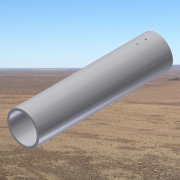
# Autodesk Inventor part: hub-sleeve
Saved by Autodesk Inventor 2013 (Build 170138000, 138)
## iProperties
Company: HERA Project
Created: 2013-05-14
Part Number: hub-sleeve
Material: PVC-Piping
Document SubType Name: Modeling
Designer: David DeBoer
Density: 1.4 g/cm^3
Mass: 429.807 g
Surface Area: 1214.86 cm^2
Volume: 307.005 cm^3
Description: Hub mating sleeve
Author: David DeBoer
Title: Hub mating sleeve
Autodesk Inventor part; units mm, degrees
ref_plane "YZ Plane" through (0, 0, 0) normal (1, 0, 0) x (0, 1, 0)
ref_plane "XZ Plane" through (0, 0, 0) normal (0, 1, 0) x (-1, 0, 0)
ref_plane "XY Plane" through (0, 0, 0) normal (0, 0, 1) x (1, 0, 0)
sketch "Sketch1" plane through (0, 0, 0) normal (0, 0, 1) x (1, 0, 0)
  circle A0 centre (0, 0) radius 36.5125
  circle A1 centre (0, 0) radius 31.3563
  dimension "d0" = 73.025
  dimension "d2" = 5.1562
  constraints: 2 centre point, 1 coincident
  measures "d0" diameter of A0
  measures "d2" radial gap between concentric circles of A1 A0
extrude "Extrusion1" add sketch "Sketch1" along normal blind 304.8
sketch "Sketch2" plane through (0, 0, 304.8) normal (0, 0, 1) x (1, 0, 0)
  circle A0 centre (0, 0) radius 31.3563 projected
  circle A1 centre (0, 0) radius 36.5125 projected
  point P0 (0, 36.5125)
  constraints: 1 vertical alignment, 1 other
ref_plane "Work Plane1" through (0, 36.5125, 304.8) normal (0, 1, 0) x (-1, 0, 0)
sketch "Sketch5" plane through (0, 36.5125, 304.8) normal (0, 1, 0) x (-1, 0, 0)
  circle A0 centre (0, -279.4) radius 4.4901
  circle A1 centre (0, -260.35) radius 4.4901
  point P0 (0, -304.8)
  dimension "d25" = 25.4
  dimension "d26" = 19.05
  constraints: 2 centre point
  measures "d25" distance of point (0, -304.8) A0.centre
  measures "d26" distance of A0.centre A1.centre
hole "Hole3" at (0, 36.5125, 44.45) at (0, 36.5125, 25.4) direction (0, -1, 0) diameter 3.175 end through all
body "Solid1"
